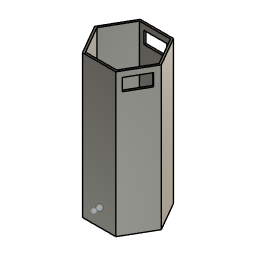
spine (Autodesk Fusion 360 design; units mm, degrees)
Autodesk Fusion 360 part; units mm, degrees
sketch "Sketch1" plane through (0, 0, 0) normal (0, 0, 1) x (1, 0, 0)
  line L0 (0, 0) -> (35, 0)
  line L1 (35, 0) -> (52.5, 30.3109)
  line L2 (52.5, 30.3109) -> (35, 60.6218)
  line L3 (35, 60.6218) -> (0, 60.6218)
  line L4 (0, 60.6218) -> (-17.5, 30.3109)
  line L5 (-17.5, 30.3109) -> (0, 0)
  point P0 (17.5, 30.3109)
  constraint coincident L0.start L5.end
extrude "Extrude1" add sketch "Sketch1" along normal blind 150
shell "Shell1" thickness 2 removed faces 2 at (11.6667, 20.2073, 0) at (11.6667, 20.2073, 150)
sketch "Sketch2" plane through (0, 60.6218, 0) normal (0, 1, 0) x (-1, 0, 0)
  line L0 (-35, 0) -> (0, 0)
  line L1 (0, 0) -> (0, 150)
  line L2 (0, 150) -> (-35, 150)
  line L3 (-35, 150) -> (-35, 0)
  line L4 (-30, 144) -> (-6, 144)
  line L5 (-6, 144) -> (-6, 131)
  line L6 (-6, 131) -> (-30, 131)
  line L7 (-30, 131) -> (-30, 144)
  constraint perpendicular L3 L4
  constraint perpendicular L2 L5
  constraint perpendicular L3 L6
  constraint perpendicular L4 L7
extrude "Extrude2" cut sketch "Sketch2" against normal blind 12 contours L4 L5 L6 L7
sketch "Sketch3" plane through (0, 0, 0) normal (0, 0, 1) x (1, 0, 0)
  line L0 (0, 12) -> (0, 18)
  constraint vertical L0
sketch "Sketch4" plane through (26.25, -15.1554, 0) normal (0.866025, -0.5, 0) x (0.5, 0.866025, 0)
  line L0 (17.5, 0) -> (52.5, 0)
  line L1 (52.5, 0) -> (52.5, 150)
  line L2 (52.5, 150) -> (17.5, 150)
  line L3 (17.5, 150) -> (17.5, 0)
  line L4 (22.5, 144) -> (46.5, 144)
  line L5 (46.5, 144) -> (46.5, 131)
  line L6 (46.5, 131) -> (22.5, 131)
  line L7 (22.5, 131) -> (22.5, 144)
  point P0 (22.5, 144)
  constraint coincident P0 L4.start
  constraint perpendicular L3 L4
  constraint perpendicular L4 L5
  constraint perpendicular L5 L6
  constraint perpendicular L4 L7
extrude "Extrude3" cut sketch "Sketch4" against normal blind 5.622 contours L4 L5 L6 L7
